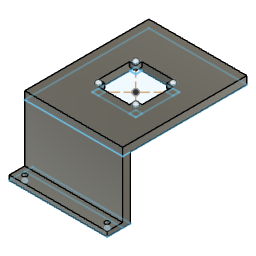
Suporte-Display v2 (Autodesk Fusion 360 design; units mm, degrees)
Autodesk Fusion 360 part; units mm, degrees
sketch "Esboço1" plane through (0, 0, 0) normal (0, 0, 1) x (1, 0, 0)
  line L0 (-50, 15) -> (13.1, 15)
  line L1 (13.1, 15) -> (13.1, 0)
  line L2 (13.1, 0) -> (-50, 0)
  line L3 (-50, 0) -> (-50, 15)
  line L4 (-50, 10) -> (13.1, 10)
  circle A0 centre (-45, 5) radius 1.5
  circle A1 centre (8.1, 5) radius 1.5
  dimension "d1" = 63.1
  dimension "d2" = 15
  dimension "d3" = 5
  dimension "d4" = 3
  dimension "d5" = 5
  dimension "d6" = 5
  dimension "d7" = 3
  dimension "d8" = 5
  dimension "d9" = 5
  constraint horizontal L0
  constraint vertical L1
  constraint horizontal L2
  constraint vertical L3
  constraint coincident L3 L4.start
  constraint coincident L1 L4.end
  constraint perpendicular L1 L4
  measures "d1" distance of L0.start L0.end
  measures "d2" distance of L0 L2
  measures "d3" distance of L0 L4
  measures "d4" diameter of A0
  measures "d5" distance of L2 A0.centre
  measures "d6" distance of L3 A0.centre
  measures "d7" diameter of A1
  measures "d8" distance of L2 A1.centre
  measures "d9" distance of L1 A1.centre
extrude "Extrusão1" add sketch "Esboço1" along normal blind 3 contours L1 L2 L3 L4
extrude "Extrusão2" add sketch "Esboço1" along normal blind 40 contours L0 L1 L3 L4
sketch "Esboço2" plane through (0, 0, 0) normal (0, 0, 1) x (1, 0, 0)
  line L0 (-50, 10, 40) -> (13.1, 10, 40)
  line L1 (13.1, 10, 40) -> (13.1, 90, 40)
  line L2 (13.1, 90, 40) -> (-50, 90, 40)
  line L3 (-50, 90, 40) -> (-50, 10, 40)
  line L4 (-32.45, 64, 40) -> (-4.45, 64, 40)
  line L5 (-4.45, 64, 40) -> (-4.45, 36, 40)
  line L6 (-4.45, 36, 40) -> (-32.45, 36, 40)
  line L7 (-32.45, 36, 40) -> (-32.45, 64, 40)
  line L8 (-32.45, 64, 40) -> (-4.45, 36, 40) construction
  line L9 (-4.45, 64, 40) -> (-32.45, 36, 40) construction
  line L10 (-32.45, 36, 40) -> (-28.45, 36, 40)
  line L11 (-28.45, 36, 40) -> (-28.45, 40, 40)
  line L12 (-28.45, 40, 40) -> (-32.45, 40, 40)
  line L13 (-32.45, 40, 40) -> (-32.45, 36, 40)
  line L14 (-32.45, 64, 40) -> (-28.45, 64, 40)
  line L15 (-28.45, 64, 40) -> (-28.45, 60, 40)
  line L16 (-28.45, 60, 40) -> (-32.45, 60, 40)
  line L17 (-32.45, 60, 40) -> (-32.45, 64, 40)
  line L18 (-4.45, 36, 40) -> (-8.45, 36, 40)
  line L19 (-8.45, 36, 40) -> (-8.45, 40.0919, 40)
  line L20 (-8.45, 40.0919, 40) -> (-4.45, 40.0919, 40)
  line L21 (-4.45, 40.0919, 40) -> (-4.45, 36, 40)
  line L22 (-4.45, 64, 40) -> (-8.45, 64, 40)
  line L23 (-8.45, 64, 40) -> (-8.45, 60, 40)
  line L24 (-8.45, 60, 40) -> (-4.45, 60, 40)
  line L25 (-4.45, 60, 40) -> (-4.45, 64, 40)
  circle A0 through (-28.95, 62, 45) (-31.2, 63.299, 45) (-31.2, 60.701, 45)
  circle A1 through (-4.95, 62, 45) (-7.2, 63.299, 45) (-7.2, 60.701, 45)
  circle A2 through (-28.95, 38, 45) (-31.2, 39.299, 45) (-31.2, 36.701, 45)
  circle A3 through (-4.95, 38.0459, 45) (-7.2, 39.345, 45) (-7.2, 36.7469, 45)
  point P0 (-18.45, 50)
  dimension "d14" = 63.1
  dimension "d15" = 80
  dimension "d17" = 28
  dimension "d18" = 28
  dimension "d19" = 4
  dimension "d20" = 4
  dimension "d21" = 4
  dimension "d22" = 4
  dimension "d23" = 4
  dimension "d24" = 4
  dimension "d25" = 4
  dimension "d34" = 3
  dimension "d35" = 3
  dimension "d36" = 3
  dimension "d37" = 3
extrude "Extrusão3" cut sketch "Esboço2" along normal blind 5 contours L0 L1 L2 L3 in plane through (0, 0, 40) normal (0, 0, 1)
extrude "Extrusão4" add sketch "Esboço2" along normal blind 5 contours L0 L1 L2 L3 in plane through (0, 0, 40) normal (0, 0, 1)
extrude "Extrusão5" add sketch "Esboço2" against normal blind 3 from surface at 5 contours L4 L7 L14 L15 L16 L17 | L4 L5 L22 L23 L24 L25 | L6 L7 L10 L11 L12 L13 | L5 L6 L18 L19 L20 L21 in plane through (0, 0, 40) normal (0, 0, 1)
hole "Furo1" at (-30.45, 38, 45) direction (0, 0, -1) diameter 3 depth 3 tip angle 118
hole "Furo2" at (-6.45, 62, 45) direction (0, 0, -1) diameter 3 depth 3 tip angle 118
hole "Furo3" at (-30.45, 62, 45) direction (0, 0, -1) diameter 3 depth 3 tip angle 118
hole "Furo4" at (-6.45, 38.0459, 45) direction (0, 0, -1) diameter 3 depth 3 tip angle 118
